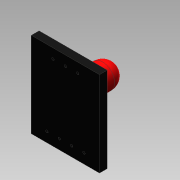
# Autodesk Inventor part: LED_module
Saved by Autodesk Inventor 2016 (Build 200138000, 138)
## iProperties
Created: 2016-05-27
Part Number: LED_module
Material: Generic
Document SubType Name: Modeling
Designer: admin
Density: 1 g/cm^3
Appearance: Glossy - Black
Mass: 0.551754 g
Surface Area: 7.23887 cm^2
Volume: 0.551754 cm^3
Author: admin
Autodesk Inventor part; units mm, degrees
ref_plane "YZ Plane" through (0, 0, 0) normal (1, 0, 0) x (0, 1, 0)
ref_plane "XZ Plane" through (0, 0, 0) normal (0, 1, 0) x (-1, 0, 0)
ref_plane "XY Plane" through (0, 0, 0) normal (0, 0, 1) x (1, 0, 0)
sketch "Sketch1" plane through (0, 0, 0) normal (0, 1, 0) x (-1, 0, 0)
  line L0 (7, 8.75) -> (-7, 8.75)
  line L1 (-7, 8.75) -> (-7, -8.75)
  line L2 (-7, -8.75) -> (7, -8.75)
  line L3 (7, -8.75) -> (7, 8.75)
  point P0 (0, 0)
  point P1 (0, -8.75)
  point P2 (-7, 0)
  dimension "d0" = 17.5
  dimension "d1" = 14
  constraints: 8 end point, 2 midpoint, 2 parallel, 1 horizontal, 1 horizontal alignment, 1 perpendicular, 1 vertical alignment
  measures "d0" distance of L2.end L0.start
  measures "d1" distance of L1.end L2.end
extrude "Extrusion1" add sketch "Sketch1" along normal blind 1.6
sketch "Sketch2" plane through (0, 1.6, 0) normal (0, 1, 0) x (1, 0, 0)
  line L0 (0, 3.5818) -> (0, 1.7058) construction
  line L1 (-7, -8.75) -> (7, -8.75) construction
  point P0 (0, 0)
  point P1 (0, -1.25)
  point P2 (-3.81, 6.75)
  point P3 (-1.27, 6.75)
  point P4 (1.27, 6.75)
  point P5 (3.81, 6.75)
  point P6 (-2.54, -6.75)
  point P7 (0, -6.75)
  point P8 (2.54, -6.75)
  dimension "d4" = 2.54
  dimension "d5" = 2.54
  dimension "d7" = 2.54
  dimension "d8" = 5.5
  dimension "d9" = 8
  dimension "d10" = 2
  constraints: 5 horizontal alignment, 3 symmetric about line, 2 end point, 2 point on line, 1 vertical, 1 vertical alignment
  measures "d4" distance of point (-1.27, 6.75) point (-3.81, 6.75)
  measures "d5" distance of point (1.27, 6.75) point (-1.27, 6.75)
  measures "d7" distance of point (0, -6.75) point (-2.54, -6.75)
  measures "d8" vertical distance of point (-2.54, -6.75) point (0, -1.25)
  measures "d9" vertical distance of point (3.81, 6.75) point (0, -1.25)
  measures "d10" distance from line of L1 point (2.54, -6.75)
hole "Hole1" at (-3.81, 1.6, -6.75) at (-1.27, 1.6, -6.75) at (1.27, 1.6, -6.75) at (3.81, 1.6, -6.75) at (-2.54, 1.6, 6.75) at (0, 1.6, 6.75) at (2.54, 1.6, 6.75) direction (0, -1, 0) diameter 0.5 end through all
sketch "Sketch3" plane through (0, 1.6, 0) normal (0, 1, 0) x (1, 0, 0)
  circle A0 centre (0, -1.25) radius 2.5
  circle A1 centre (0, -6.75) radius 0.25 projected
  point P0 (0, 0)
  dimension "d20" = 5.5
  dimension "d21" = 5
  constraints: 1 centre point, 1 vertical alignment
  measures "d20" distance of A0.centre A1.centre
  measures "d21" diameter of A0
sketch "Sketch4" plane through (0, 1.6, 0) normal (0, 1, 0) x (1, 0, 0)
  point P0 (0, 0)
extrude "Extrusion2" add sketch "Sketch3" along normal blind 8.5 contours A0
fillet "Fillet1" radius 2.5 1 edges at (-2.5, 10.1, 1.25)
sketch "Sketch5" plane through (0, 1.6, 0) normal (0, 1, 0) x (1, 0, 0)
  circle A0 centre (0, -1.25) radius 2.5 projected
  arc A1 (-2.5, -3.3267) -> (-2.5, 0.8267) centre (0, -1.25) ccw
  line L0 (-2.5, 0.8267) -> (-2.5, -3.3267)
  point P0 (0, 0)
  point P1 (-2.5, -1.25)
  dimension "d23" = 6.5
  constraints: 2 end point, 2 point on circle, 1 centre point, 1 coincident, 1 horizontal alignment, 1 midpoint, 1 vertical, 1 other
  measures "d23" diameter of A1
extrude "Extrusion3" add sketch "Sketch5" along normal blind 1
equation "\"d5\" = d4"
equation "\"d7\" = d4"
body "Solid1"
